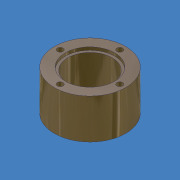
# Autodesk Inventor part: BB1-RingGear
Saved by Autodesk Inventor 2015 (Build 190159000, 159)
## iProperties
Company: FirstCadLibrary
Shininess: 64.0
Length Units: 11269
Angle Units: 11279
Time Units: 11290
Mass Units: 11283
Length Display Precision: 3
Angle Display Precision: 2
Compacted: True
Part Number: BB1-RingGear
Document SubType Name: Modeling
Created: 2007-01-08
Material: Aluminum-6061
Designer: Ed Sparks
Catalog Web Link: www.banebots.com
Vendor: BaneBots
Density: 1 g/cm^3
Appearance: Gunmetal - Antique Polished
Density: 0.0
Volumn: 0.0
Area: 0.0
PropertySet Name: Model Information
Control State: 0
Master: False
Checked Out: False
Author: Ed Sparks
Autodesk Inventor part; units mm, degrees
ref_plane "YZ Plane" through (0, 0, 0) normal (1, 0, 0) x (0, 1, 0)
ref_plane "XZ Plane" through (0, 0, 0) normal (0, 1, 0) x (-1, 0, 0)
ref_plane "XY Plane" through (0, 0, 0) normal (0, 0, 1) x (1, 0, 0)
sketch "Sketch1" plane through (0, 0, 0) normal (0, 0, 1) x (1, 0, 0)
  circle A0 centre (0, 0) radius 20.9
  circle A1 centre (0, 0) radius 13
  dimension "d0" = 41.8
  dimension "d1" = 26
  constraints: 2 centre point, 2 coincident, 1 concentric, 1 other
  measures "d0" diameter of A0
  measures "d1" diameter of A1
extrude "Extrusion1" add sketch "Sketch1" along normal mid plane 23.368
sketch "Sketch2" plane through (0, 0, 11.684) normal (0, 0, 1) x (1, 0, 0)
  circle A0 centre (0, 0) radius 13 projected
  point P0 (0, 17.5)
  dimension "d4" = 17.5
  constraints: 1 vertical alignment
  measures "d4" distance of point (0, 17.5) A0.centre
hole "Hole1" at (0, 17.5, 11.684) direction (0, 0, -1) diameter 3.5 end through all
pattern_circular "Circular Pattern1" count 4 over 360 about axis through (0, 0, 0) along (0, 0, 1) of "Hole1"
sketch "Sketch3" plane through (0, 0, 11.684) normal (0, 0, 1) x (1, 0, 0)
  circle A0 centre (0, 0) radius 13 projected
  circle A1 centre (0, 0) radius 20.9 projected
  circle A2 centre (0, 0) radius 14.5
  dimension "d15" = 29
  constraints: 1 centre point, 1 coincident, 1 concentric
  measures "d15" diameter of A2
extrude "Extrusion2" cut sketch "Sketch3" against normal blind 1.75 contours A2
mirror "Mirror1" about plane through (0, 0, 0) normal (0, 0, 1) of "Extrusion2"
body "Solid1"
